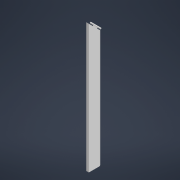
# Autodesk Inventor part: frame
Saved by Autodesk Inventor 2021 (Build 250183000, 183)
## iProperties
Created: 2020-05-07
Part Number: frame
Material: Generic
Document SubType Name: Modeling
Designer: Jonathan
Density: 1 g/cm^3
Appearance: Default
Author: Jonathan
Autodesk Inventor part; units mm, degrees
ref_plane "YZ Plane" through (0, 0, 0) normal (1, 0, 0) x (0, 1, 0)
ref_plane "XZ Plane" through (0, 0, 0) normal (0, 1, 0) x (-1, 0, 0)
ref_plane "XY Plane" through (0, 0, 0) normal (0, 0, 1) x (1, 0, 0)
sketch "Sketch1" plane through (0, 0, 0) normal (0, 1, 0) x (-1, 0, 0)
  line L0 (5, 0) -> (25, 0)
  line L1 (25, 0) -> (0, 0)
  line L2 (0, 5) -> (0, 25)
  line L3 (25, 0) -> (25, 5)
  line L4 (25, 5) -> (10, 5)
  line L5 (5, 10) -> (5, 25)
  line L6 (5, 25) -> (0, 25)
  arc A0 (0, 5) -> (5, 0) centre (5, 5) ccw
  arc A1 (5, 10) -> (10, 5) centre (10, 10) ccw
  dimension "d0" = 25
  dimension "d1" = 5
  dimension "d8" = 5
  constraints: 14 end point, 5 perpendicular, 4 point on circle, 4 tangent, 2 centre point, 2 point on line, 2 vertical, 1 collinear, 1 equal radius, 1 horizontal
  measures "d0" distance of L1.end L0.end
  measures "d1" radius of A0
  measures "d8" distance of L5.end L2.end
extrude "Extrusion1" add sketch "Sketch1" along normal blind 250
sketch "Sketch3" plane through (0, 0, 25) normal (1, 0, 0) x (0, 0, -1)
  line L0 (0, 250) -> (25, 225)
  line L1 (0, 250) -> (20, 250) projected
  line L2 (25, 250) -> (20, 250) projected
  line L3 (25, 0) -> (25, 250) projected
  dimension "d5" = 45
  constraints: 2 end point, 1 coincident
  measures "d5" angle of L1 L0
extrude "Extrusion2" cut sketch "Sketch3" against normal through all
sketch "Sketch4" plane through (-25, 0, 0) normal (-1, 0, 0) x (0, 0, 1)
  circle A0 centre (-3.1066, 225.2782) radius 1.5 construction
  circle A1 centre (-3.1066, 225.2782) radius 1.3
  point P0 (0, 0)
  dimension "d9" = 0.2
  constraints: 1 centre point
  measures "d9" radial gap between concentric circles of A0 A1
ref_plane "Work Plane1" through (-5, 221.7426, -7.0711) normal (1, 0, 0) x (0, 0.7071068, 0.7071068)
extrude "Extrusion3" add sketch "Sketch4" against normal up to surface (20 mm away)
sketch "Sketch5" plane through (-25, 225.2782, -3.1066) normal (-1, 0, 0) x (0, 0, 1)
  circle A0 centre (0, 0) radius 1.3 projected
  line L0 (3.1066, -225.2782) -> (3.1066, -0.2782) projected
  line L1 (1.0607, 1.0607) -> (2.4749, -0.3536) construction
  line L2 (3.1066, -0.2782) -> (0.6451, 1.1287)
  line L3 (3.1066, -9.7382) -> (-1.1782, -0.5494)
  line L4 (3.1066, -9.7382) -> (3.1066, -0.2782)
  point P0 (1.2627, 0.3093)
  point P1 (3.1066, -1.5346)
  point P2 (3.1066, -9.7042)
  dimension "d20" = 25
  constraints: 6 end point, 3 point on circle, 3 point on line, 2 tangent, 1 collinear
  measures "d20" angle of L0 L3
ref_plane "Work Plane2" through (-18.3333, 221.157, -6.5207) normal (1, 0, 0) x (0, 0.7071068, -0.7071068)
ref_plane "Work Plane3" through (-11.6667, 221.157, -6.5207) normal (-1, 0, 0) x (0, 0.7071068, 0.7071068)
extrude "Extrusion4" add sketch "Sketch5" against normal up to surface (6.6667 mm away) from surface at -6.6667
sketch "Sketch6" plane through (-18.3333, 215.8282, 0) normal (-1, 0, 0) x (0, 0, 1)
  arc A0 (-4.2848, 8.9006) -> (-2.4615, 10.5787) centre (-3.1066, 9.45) ccw projected
  line L0 (0, 9.1718) -> (0, -0.2882) projected
  line L1 (-4.2848, 8.9006) -> (0, -0.2882) projected
  line L2 (0, 9.1718) -> (-2.4615, 10.5787) projected
  point P0 (0, -215.8282)
extrude "Extrusion5" cut sketch "Sketch6" against normal blind 0.3
sketch "Sketch7" plane through (-11.6667, 215.8282, 0) normal (1, 0, 0) x (0, 0, -1)
  line L0 (0, -0.2882) -> (0, 9.1718) projected
  arc A0 (2.4615, 10.5787) -> (4.2848, 8.9006) centre (3.1066, 9.45) ccw projected
  line L1 (2.4615, 10.5787) -> (0, 9.1718) projected
  line L2 (0, -0.2882) -> (4.2848, 8.9006) projected
  point P0 (0, -215.8282)
extrude "Extrusion6" cut sketch "Sketch7" against normal blind 0.3
body "Solid1"
